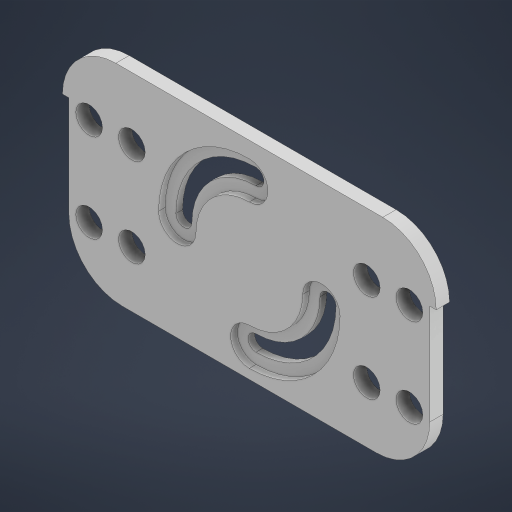
# Autodesk Inventor part: Back_plate
Saved by Autodesk Inventor 2024 (Build 280153000, 153)
## iProperties
Created: 2024-02-08
Part Number: Back_plate
Material: Generic
Document SubType Name: Modeling
Designer: calvi
Density: 1 g/cm^3
Appearance: Default
Author: calvi
Autodesk Inventor part; units mm, degrees
ref_plane "YZ Plane" through (0, 0, 0) normal (1, 0, 0) x (0, 1, 0)
ref_plane "XZ Plane" through (0, 0, 0) normal (0, 1, 0) x (-1, 0, 0)
ref_plane "XY Plane" through (0, 0, 0) normal (0, 0, 1) x (1, 0, 0)
sketch "Sketch1" plane through (0, 0, 0) normal (0, 0, 1) x (1, 0, 0)
  line L0 (0, 0) -> (177.8, 0)
  line L1 (177.8, 0) -> (177.8, 101.6)
  line L2 (177.8, 101.6) -> (0, 101.6)
  line L3 (0, 101.6) -> (0, 0)
  arc A0 (25.4, 101.6) -> (0, 76.2) centre (25.4, 76.2) ccw
  arc A1 (177.8, 76.2) -> (152.4, 101.6) centre (152.4, 76.2) ccw
  arc A2 (152.4, 0) -> (177.8, 25.4) centre (152.4, 25.4) ccw
  arc A3 (0, 25.4) -> (25.4, 0) centre (25.4, 25.4) ccw
  arc A4 (88.9, 85.09) -> (54.61, 50.8) centre (88.9, 50.8) ccw construction
  arc A5 (88.9, 88.9) -> (50.8, 50.8) centre (88.9, 50.8) ccw
  arc A6 (88.9, 81.28) -> (58.42, 50.8) centre (88.9, 50.8) ccw
  arc A7 (88.9, 81.28) -> (88.9, 88.9) centre (88.9, 85.09) ccw
  arc A8 (50.8, 50.8) -> (58.42, 50.8) centre (54.61, 50.8) ccw
  line L4 (88.9, 50.8) -> (54.61, 50.8) construction
  line L5 (88.9, 50.8) -> (88.9, 85.09) construction
  arc A9 (88.9, 20.32) -> (119.38, 50.8) centre (88.9, 50.8) ccw
  line L6 (88.9, 50.8) -> (123.19, 50.8) construction
  arc A10 (88.9, 16.51) -> (123.19, 50.8) centre (88.9, 50.8) ccw construction
  arc A11 (127, 50.8) -> (119.38, 50.8) centre (123.19, 50.8) ccw
  arc A12 (88.9, 12.7) -> (127, 50.8) centre (88.9, 50.8) ccw
  arc A13 (88.9, 20.32) -> (88.9, 12.7) centre (88.9, 16.51) ccw
  line L7 (0, 50.8) -> (177.8, 50.8)
  line L8 (88.9, 101.6) -> (88.9, 0)
  circle A14 centre (12.7, 71.882) radius 6.35
  circle A15 centre (33.02, 71.882) radius 6.35
  circle A16 centre (12.7, 29.718) radius 6.35
  circle A17 centre (33.02, 29.718) radius 6.35
  circle A18 centre (165.1, 29.718) radius 6.35
  circle A19 centre (144.78, 29.718) radius 6.35
  circle A20 centre (165.1, 71.882) radius 6.35
  circle A21 centre (144.78, 71.882) radius 6.35
  point P0 (0, 0)
  point P1 (0, 0)
  point P2 (-19.4884, -65.4138)
  dimension "d2" = 177.8
  dimension "d3" = 101.6
  dimension "d4" = 50.8
  dimension "d5" = 50.8
  dimension "d6" = 50.8
  dimension "d7" = 50.8
  dimension "d9" = 50.8
  dimension "d10" = 88.9
  dimension "d11" = 34.29
  dimension "d12" = 90
  dimension "d13" = 7.62
  dimension "d14" = 360
  dimension "d15" = 0
  dimension "d16" = 0
  dimension "d17" = 0
  dimension "d19" = 0
  dimension "d20" = 12.7
  dimension "d21" = 12.7
  dimension "d22" = 20.32
  dimension "d24" = 21.082
  dimension "d25" = 12.7
  constraints: 28 point on circle, 22 centre point, 18 end point, 12 tangent, 8 point on line, 6 symmetric about line, 4 midpoint, 2 parallel, 2 perpendicular, 2 vertical, 1 coincident, 1 horizontal, 1 horizontal alignment, 33 other
  measures "d2" distance of L2.end L1.end
  measures "d3" distance of L1.end L0.end
  measures "d4" diameter of A0
  measures "d5" diameter of A1
  measures "d6" diameter of A2
  measures "d7" diameter of A3
  measures "d9" distance from line of L0 point (88.9, 50.8)
  measures "d10" distance from line of L1 point (88.9, 50.8)
  measures "d11" radius of A4
  measures "d12" angle of L5 L4
  measures "d13" diameter of A8
  measures "d15" distance of point (0, 0) L0.start
  measures "d16" distance of L0.start point (0, 0)
  measures "d17" distance of point (0, 0) point (0, 0)
  measures "d19" distance of point (0, 0) point (0, 0)
  measures "d20" diameter of A14
  measures "d21" diameter of A15
  measures "d22" distance of A15.centre A14.centre
  measures "d24" distance from line of L7 A14.centre
  measures "d25" distance from line of L3 A14.centre
extrude "Extrusion1" add sketch "Sketch1" along normal blind 3.175 contours A3 L3 L7 A8 L8 A13 L0 | L8 A12 L7 L1 A2 L0 | L3 A0 L2 L8 A5 L7 | A11 L7 L8 A7 L2 A1 L1 | L8 L7 A9 | A6 L8 L7
sketch "Sketch2" plane through (0, 0, 3.175) normal (0, 0, 1) x (1, 0, 0)
  line L0 (0, 0) -> (177.8, 0)
  line L1 (177.8, 0) -> (177.8, 101.6)
  line L2 (177.8, 101.6) -> (0, 101.6)
  line L3 (0, 101.6) -> (0, 0)
  circle A0 centre (12.7, 71.882) radius 6.35
  circle A1 centre (12.7, 71.882) radius 6.35 projected
  circle A2 centre (33.02, 71.882) radius 6.35
  circle A3 centre (12.7, 29.718) radius 6.35
  circle A4 centre (33.02, 29.718) radius 6.35
  circle A5 centre (33.02, 71.882) radius 6.35 projected
  circle A6 centre (12.7, 29.718) radius 6.35 projected
  circle A7 centre (33.02, 29.718) radius 6.35 projected
  circle A8 centre (144.78, 71.882) radius 6.35
  circle A9 centre (144.78, 29.718) radius 6.35
  circle A10 centre (165.1, 71.882) radius 6.35
  circle A11 centre (165.1, 29.718) radius 6.35
  circle A12 centre (144.78, 71.882) radius 6.35 projected
  circle A13 centre (165.1, 71.882) radius 6.35 projected
  circle A14 centre (144.78, 29.718) radius 6.35 projected
  circle A15 centre (165.1, 29.718) radius 6.35 projected
  arc A16 (88.9, 85.09) -> (54.61, 50.8) centre (88.9, 50.8) ccw construction
  arc A17 (88.9, 93.98) -> (45.72, 50.8) centre (88.9, 50.8) ccw
  arc A18 (88.9, 76.2) -> (63.5, 50.8) centre (88.9, 50.8) ccw
  arc A19 (88.9, 76.2) -> (88.9, 93.98) centre (88.9, 85.09) ccw
  arc A20 (45.72, 50.8) -> (63.5, 50.8) centre (54.61, 50.8) ccw
  line L4 (88.9, 50.8) -> (54.61, 50.8) construction
  line L5 (88.9, 50.8) -> (88.9, 85.09) construction
  arc A21 (88.9, 25.4) -> (114.3, 50.8) centre (88.9, 50.8) ccw
  line L6 (88.9, 50.8) -> (123.19, 50.8) construction
  arc A22 (88.9, 16.51) -> (123.19, 50.8) centre (88.9, 50.8) ccw construction
  arc A23 (88.9, 7.62) -> (132.08, 50.8) centre (88.9, 50.8) ccw
  arc A24 (132.08, 50.8) -> (114.3, 50.8) centre (123.19, 50.8) ccw
  arc A25 (88.9, 25.4) -> (88.9, 7.62) centre (88.9, 16.51) ccw
  arc A26 (25.4, 101.6) -> (0, 76.2) centre (25.4, 76.2) ccw
  arc A27 (0, 25.4) -> (25.4, 0) centre (25.4, 25.4) ccw
  line L7 (177.8, 25.4) -> (177.8, 76.2) projected
  arc A28 (152.4, 0) -> (177.8, 25.4) centre (152.4, 25.4) ccw
  arc A29 (129.8378, 37.0665) -> (128.016, 32.512) centre (152.4, 25.4) ccw
  arc A30 (177.8, 76.2) -> (152.4, 101.6) centre (152.4, 76.2) ccw
  arc A31 (177.8, 76.2) -> (152.4, 101.6) centre (152.4, 76.2) ccw projected
  dimension "d28" = 177.8
  dimension "d29" = 101.6
  dimension "d30" = 12.7
  dimension "d31" = 12.7
  dimension "d32" = 12.7
  dimension "d33" = 12.7
  dimension "d34" = 12.7
  dimension "d35" = 12.7
  dimension "d36" = 12.7
  dimension "d37" = 12.7
  dimension "d38" = 34.29
  dimension "d39" = 90
  dimension "d40" = 17.78
  dimension "d41" = 50.8
  dimension "d42" = 88.9
  dimension "d45" = 360
  dimension "d48" = 25.4
  dimension "d49" = 50.8
  dimension "d57" = 50.8
  constraints: 31 point on circle, 23 centre point, 15 end point, 10 tangent, 9 concentric, 7 point on line, 2 coincident, 2 parallel, 1 horizontal, 1 perpendicular, 25 other
  measures "d28" distance of L2.end L1.end
  measures "d29" distance of L1.end L0.end
  measures "d30" diameter of A0
  measures "d31" diameter of A2
  measures "d32" diameter of A3
  measures "d33" diameter of A4
  measures "d34" diameter of A8
  measures "d35" diameter of A9
  measures "d36" diameter of A10
  measures "d37" diameter of A11
  measures "d38" radius of A16
  measures "d39" angle of L5 L4
  measures "d40" diameter of A20
  measures "d41" distance from line of L0 L4.start
  measures "d42" distance between parallel lines of L3 L5
  measures "d48" distance from line of L2 A26.centre
  measures "d49" diameter of A27
  measures "d57" diameter of A30
extrude "Extrusion2" add sketch "Sketch2" along normal blind 3.175 contours A27 L3 A26 L2 A30 L1 A28 L0
sketch "Sketch3" plane through (177.8, 25.4, 0) normal (1, 0, 0) x (0, 0, -1)
  line L0 (-6.35, 0) -> (-6.35, 50.8) projected
  line L1 (-6.35, 50.8) -> (0, 50.8)
  line L2 (0, 50.8) -> (0, -25.4)
  line L3 (0, -25.4) -> (-6.35, -25.4)
  line L4 (-6.35, -25.4) -> (-6.35, 50.8)
  constraints: 8 end point, 2 parallel, 1 horizontal, 1 perpendicular
extrude "Extrusion3" cut sketch "Sketch3" against normal blind 3.048
sketch "Sketch4" plane through (0, 25.4, 0) normal (-1, 0, 0) x (0, 0, 1)
  line L0 (6.35, 50.8) -> (0, 50.8) projected
  line L1 (6.35, -25.4) -> (6.35, 0) projected
  line L2 (0, 50.8) -> (6.35, 50.8)
  line L3 (6.35, 50.8) -> (6.35, -25.4)
  line L4 (6.35, -25.4) -> (0, -25.4)
  line L5 (0, -25.4) -> (0, 50.8)
  point P0 (0, -25.4)
  constraints: 8 end point, 2 parallel, 1 horizontal, 1 perpendicular
extrude "Extrusion4" cut sketch "Sketch4" against normal blind 3.048
sketch "Sketch5" plane through (25.4, 0, 0) normal (0, -1, 0) x (1, 0, 0)
  line L0 (-22.352, 6.35) -> (-22.352, 0) projected
  line L1 (149.352, 6.35) -> (149.352, 0) projected
  line L2 (-22.352, 6.35) -> (149.352, 6.35)
  line L3 (149.352, 6.35) -> (149.352, 0)
  line L4 (149.352, 0) -> (-22.352, 0)
  line L5 (-22.352, 0) -> (-22.352, 6.35)
  point P0 (-25.4, 0)
  constraints: 8 end point, 2 parallel, 1 horizontal, 1 perpendicular
extrude "Extrusion5" cut sketch "Sketch5" against normal blind 3.048
sketch "Sketch6" plane through (0, 0, 6.35) normal (0, 0, 1) x (1, 0, 0)
  arc A0 (3.048, 28.448) -> (28.448, 3.048) centre (28.448, 28.448) ccw
  arc A1 (149.352, 3.048) -> (174.752, 28.448) centre (149.352, 28.448) ccw
  line L0 (3.048, 76.2) -> (3.048, 13.3357) projected
  line L1 (13.3357, 3.048) -> (164.4643, 3.048) projected
  line L2 (174.752, 13.3357) -> (174.752, 76.2) projected
  line L3 (3.048, 28.448) -> (3.048, 3.048)
  line L4 (3.048, 3.048) -> (28.448, 3.048)
  line L5 (174.752, 28.448) -> (174.752, 3.048)
  line L6 (149.352, 3.048) -> (174.752, 3.048)
  point P0 (0, 0)
  point P1 (3.048, 13.3357)
  dimension "d66" = 50.8
  dimension "d67" = 50.8
  constraints: 8 end point, 7 point on line, 6 tangent, 4 point on circle, 2 centre point, 1 perpendicular
  measures "d66" diameter of A0
  measures "d67" diameter of A1
extrude "Extrusion6" cut sketch "Sketch6" against normal through all
body "Solid1"
